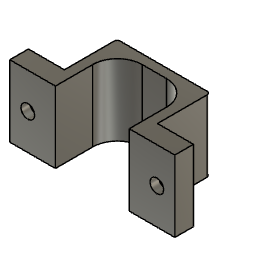
fixation moteur N20 v3 (Autodesk Fusion 360 design; units mm, degrees)
Autodesk Fusion 360 part; units mm, degrees
sketch "Sketch1" plane through (0, 0, 0) normal (0, 0, 1) x (1, 0, 0)
  line L0 (-13.3, 0) -> (-13.3, 3)
  line L1 (-13.3, 3) -> (-7.5, 3)
  line L2 (-7.5, 3) -> (-7.5, 11.5)
  line L3 (-7.5, 11.5) -> (0, 11.5)
  line L4 (-13.3, 0) -> (-5.95, 0)
  line L5 (-5.95, 0) -> (-5.95, 10)
  line L6 (-5.95, 10) -> (0, 10)
  line L7 (0, 0) -> (0, 65)
  line L8 (7.5, 3) -> (7.5, 11.5)
  line L9 (13.3, 0) -> (13.3, 3)
  line L10 (5.95, 0) -> (5.95, 10)
  line L11 (13.3, 0) -> (5.95, 0)
  line L12 (13.3, 3) -> (7.5, 3)
  line L13 (5.95, 10) -> (0, 10)
  line L14 (7.5, 11.5) -> (0, 11.5)
  dimension "d1" = 11.9
  dimension "d2" = 15
  dimension "d3" = 26.6
  dimension "d4" = 10
  dimension "d5" = 11.5
  dimension "d6" = 3
  constraint vertical L0
  constraint perpendicular L0 L1
  constraint perpendicular L1 L2
  constraint perpendicular L2 L3
  constraint perpendicular L0 L4
  constraint perpendicular L4 L5
  constraint perpendicular L5 L6
  constraint coincident L7.start origin
  constraint perpendicular L3 L7
  constraint symmetric origin L7 L7.start
  constraint symmetric L0.start L7 L9.start
  constraint symmetric L0.end L7 L9.end
  constraint symmetric L1.end L7 L8.start
  constraint symmetric L2.end L7 L8.end
  constraint symmetric L3.end L7 L14.end
  constraint symmetric L4.end L7 L10.start
  constraint symmetric L5.end L7 L10.end
  constraint symmetric L6.end L7 L13.end
  measures "d1" distance of L5 L10
  measures "d2" distance of L2 L8
  measures "d3" distance of L0 L9
  measures "d4" distance of L11 L13
  measures "d5" distance of L11 L14
  measures "d6" distance of L11 L12
extrude "Extrude1" add sketch "Sketch1" along normal blind 11.5
fillet "Fillet1" radius 0.5 1 edges at (7.5, 11.5, 5.75)
fillet "Fillet2" radius 0.5 1 edges at (-7.5, 11.5, 5.75)
fillet "Fillet3" radius 4 1 edges at (-5.95, 10, 5.75)
fillet "Fillet4" radius 4 1 edges at (5.95, 10, 5.75)
sketch "Sketch2" plane through (0, 3, 0) normal (0, 1, 0) x (-1, 0, 0)
  line L0 (7.5, 0) -> (13.3, 0)
  line L1 (13.3, 0) -> (13.3, 11.5)
  line L2 (13.3, 11.5) -> (7.5, 11.5)
  line L3 (7.5, 11.5) -> (7.5, 0)
  line L4 (7.5, 11.5) -> (13.3, 0) construction
  line L5 (13.3, 11.5) -> (7.5, 0) construction
  circle A0 centre (10.4, 5.75) radius 2.35 construction
  arc A1 (11.4582, 7.8482) -> (9.112, 7.7156) centre (10.4, 5.75) ccw construction
  line L6 (10.4, 5.75) -> (11.4582, 7.8482) construction
  line L7 (10.4, 5.75) -> (9.112, 7.7156) construction
  line L8 (11.4582, 7.8482) -> (9.112, 7.7156)
  line L9 (8.0537, 5.6173) -> (9.112, 7.7156)
  line L10 (11.688, 3.7844) -> (12.7463, 5.8827)
  line L11 (11.4582, 7.8482) -> (12.7463, 5.8827)
  line L12 (8.0537, 5.6173) -> (9.3418, 3.6518)
  line L13 (9.3418, 3.6518) -> (11.688, 3.7844)
  line L14 (0, 0) -> (0, 11.4709) construction
  line L15 (-11.4582, 7.8482) -> (-9.112, 7.7156)
  line L16 (-11.688, 3.7844) -> (-12.7463, 5.8827)
  line L17 (-11.4582, 7.8482) -> (-12.7463, 5.8827)
  line L18 (-9.3418, 3.6518) -> (-11.688, 3.7844)
  line L19 (-8.0537, 5.6173) -> (-9.3418, 3.6518)
  line L20 (-8.0537, 5.6173) -> (-9.112, 7.7156)
  dimension "d17" = 4.7
  dimension "d18" = 60
  constraint coincident L2.end L3.start
  constraint coincident L0.end L1.start
  constraint coincident L1.end L2.start
  constraint coincident L0.start L3.end
  constraint midpoint L5 A0.centre
  constraint coincident A0 A1.start
  constraint coincident L5 A1.start
  constraint coincident A0.centre A1.centre
  constraint symmetric A1.start L7 L9.start
  constraint symmetric A1.end L7 L8.end
  constraint symmetric A1.start L6 L8.start
  constraint symmetric A1.end L6 L10.end
  constraint symmetric L6 L9.start L10.start
  constraint symmetric L6 A1.end L10.end
  constraint coincident L5 L12.end
  constraint coincident A0 L12.end
  constraint coincident L14.start origin
  constraint parallel L1 L14
  constraint symmetric A1.start L14 L15.start
  constraint symmetric A1.end L14 L15.end
  constraint symmetric L9.start L14 L19.start
  constraint symmetric L10.start L14 L16.start
  constraint symmetric L10.end L14 L16.end
  constraint symmetric L12.end L14 L18.start
  measures "d17" diameter of A0
  measures "d18" angle of L6 L7
extrude "Extrude2" cut sketch "Sketch2" against normal blind 1.6 contours L8 L9 L10 L11 L12 L13 | L15 L16 L17 L18 L19 L20
sketch "Sketch3" plane through (0, 1.4, 0) normal (0, 1, 0) x (-1, 0, 0)
  line L0 (8.0537, 5.6173) -> (9.3418, 3.6518)
  line L1 (9.3418, 3.6518) -> (11.688, 3.7844)
  line L2 (11.688, 3.7844) -> (12.7463, 5.8827)
  line L3 (12.7463, 5.8827) -> (11.4582, 7.8482)
  line L4 (11.4582, 7.8482) -> (9.112, 7.7156)
  line L5 (9.112, 7.7156) -> (8.0537, 5.6173)
  line L6 (9.112, 7.7156) -> (11.688, 3.7844) construction
  line L7 (11.4582, 7.8482) -> (9.3418, 3.6518) construction
  circle A0 centre (10.4, 5.75) radius 1.1
  line L8 (0, 0) -> (0, 11.5) construction
  circle A1 centre (-10.4, 5.75) radius 1.1
  dimension "d21" = 2.2
  constraint coincident L4.end L5.start
  constraint coincident L1.end L2.start
  constraint coincident L3.end L4.start
  constraint coincident L0.end L1.start
  constraint midpoint L7 A0.centre
  constraint coincident L8.start origin
  constraint vertical L8
  constraint symmetric A0 L8 A1
  measures "d21" diameter of A0
extrude "Extrude3" cut sketch "Sketch3" against normal blind 1.8 contours A0 | A1
